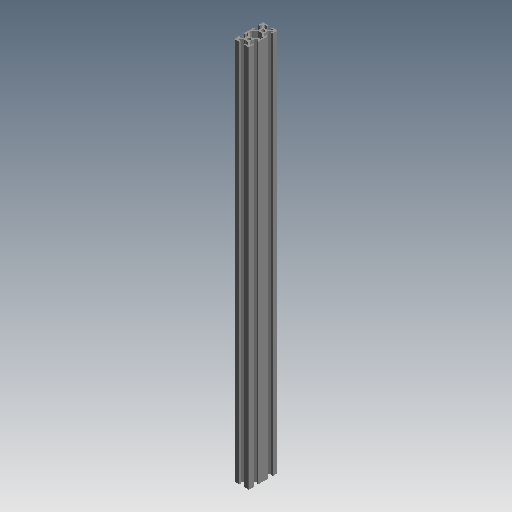
# Autodesk Inventor part: HFS5-2040-530
Saved by Autodesk Inventor 2020 (Build 240168000, 168)
## iProperties
Part Number: HFS5-2040-530
Material: Generic
Catalog Web Link: www.cadenas.de
Description: NFS5-2040, NFSB5-2040, HFS5-2040, HFSB5-2040, CAF5-2040, NFSF5-2040, HFSF5-2040-HFS5 Series Aluminum Extrusions 20,40 Square -2 Slots-
Vendor: MISUMI
Document SubType Name: Modeling
Designer: partserver
Manufacturer: MISUMI
Mass: 171.584 g
Surface Area: 1671.65 cm^2
Volume: 171.584 cm^3
Density: 1 g/cm^3
Appearance: PSOLRGB-175-175-175
Category: PARTsolutions
Company: MISUMI
Title: HFS5-2040-530
Author: Cadenas PARTsolutions
Comments: HFS5 Series Aluminum Extrusions 20,40 Square -2 Slots-
Autodesk Inventor part; units mm, degrees
sketch "Sketch_1" plane through (0, 0, 0) normal (0, 0, 1) x (1, 0, 0)
  line L0 (-10, -7) -> (-8, -7)
  line L1 (-8, -7) -> (-8, -4)
  line L2 (-8, -4) -> (-7.0607, -4)
  line L3 (-7.0607, -4) -> (-4, -7.0607)
  line L4 (-4, -7.0607) -> (-4, -9.4804)
  line L5 (-4, -9.4804) -> (-3.7, -10)
  line L6 (-3.7, -10) -> (-4, -10.5196)
  line L7 (-4, -10.5196) -> (-4, -12.9393)
  line L8 (-4, -12.9393) -> (-7.0607, -16)
  line L9 (-7.0607, -16) -> (-8, -16)
  line L10 (-8, -16) -> (-8, -13)
  line L11 (-8, -13) -> (-10, -13)
  line L12 (-10, -13) -> (-10, -19)
  arc A0 (-10, -19) -> (-9, -20) centre (-9, -19) ccw
  line L13 (-9, -20) -> (-3, -20)
  line L14 (-3, -20) -> (-3, -18)
  line L15 (-3, -18) -> (-6, -18)
  line L16 (-6, -18) -> (-6, -17.0607)
  line L17 (-6, -17.0607) -> (-2.9393, -14)
  line L18 (-2.9393, -14) -> (-0.5196, -14)
  line L19 (-0.5196, -14) -> (0, -13.7)
  line L20 (0, -13.7) -> (0.5196, -14)
  line L21 (0.5196, -14) -> (2.9393, -14)
  line L22 (2.9393, -14) -> (6, -17.0607)
  line L23 (6, -17.0607) -> (6, -18)
  line L24 (6, -18) -> (3, -18)
  line L25 (3, -18) -> (3, -20)
  line L26 (3, -20) -> (9, -20)
  arc A1 (9, -20) -> (10, -19) centre (9, -19) ccw
  line L27 (10, -19) -> (10, -13)
  line L28 (10, -13) -> (8, -13)
  line L29 (8, -13) -> (8, -16)
  line L30 (8, -16) -> (7.0607, -16)
  line L31 (7.0607, -16) -> (4, -12.9393)
  line L32 (4, -12.9393) -> (4, -10.5196)
  line L33 (4, -10.5196) -> (3.7, -10)
  line L34 (3.7, -10) -> (4, -9.4804)
  line L35 (4, -9.4804) -> (4, -7.0607)
  line L36 (4, -7.0607) -> (7.0607, -4)
  line L37 (7.0607, -4) -> (8, -4)
  line L38 (8, -4) -> (8, -7)
  line L39 (8, -7) -> (10, -7)
  line L40 (10, -7) -> (10, 7)
  line L41 (10, 7) -> (8, 7)
  line L42 (8, 7) -> (8, 4)
  line L43 (8, 4) -> (7.0607, 4)
  line L44 (7.0607, 4) -> (4, 7.0607)
  line L45 (4, 7.0607) -> (4, 9.4804)
  line L46 (4, 9.4804) -> (3.7, 10)
  line L47 (3.7, 10) -> (4, 10.5196)
  line L48 (4, 10.5196) -> (4, 12.9393)
  line L49 (4, 12.9393) -> (7.0607, 16)
  line L50 (7.0607, 16) -> (8, 16)
  line L51 (8, 16) -> (8, 13)
  line L52 (8, 13) -> (10, 13)
  line L53 (10, 13) -> (10, 19)
  arc A2 (10, 19) -> (9, 20) centre (9, 19) ccw
  line L54 (9, 20) -> (3, 20)
  line L55 (3, 20) -> (3, 18)
  line L56 (3, 18) -> (6, 18)
  line L57 (6, 18) -> (6, 17.0607)
  line L58 (6, 17.0607) -> (2.9393, 14)
  line L59 (2.9393, 14) -> (0.5196, 14)
  line L60 (0.5196, 14) -> (0, 13.7)
  line L61 (0, 13.7) -> (-0.5196, 14)
  line L62 (-0.5196, 14) -> (-2.9393, 14)
  line L63 (-2.9393, 14) -> (-6, 17.0607)
  line L64 (-6, 17.0607) -> (-6, 18)
  line L65 (-6, 18) -> (-3, 18)
  line L66 (-3, 18) -> (-3, 20)
  line L67 (-3, 20) -> (-9, 20)
  arc A3 (-9, 20) -> (-10, 19) centre (-9, 19) ccw
  line L68 (-10, 19) -> (-10, 13)
  line L69 (-10, 13) -> (-8, 13)
  line L70 (-8, 13) -> (-8, 16)
  line L71 (-8, 16) -> (-7.0607, 16)
  line L72 (-7.0607, 16) -> (-4, 12.9393)
  line L73 (-4, 12.9393) -> (-4, 10.5196)
  line L74 (-4, 10.5196) -> (-3.7, 10)
  line L75 (-3.7, 10) -> (-4, 9.4804)
  line L76 (-4, 9.4804) -> (-4, 7.0607)
  line L77 (-4, 7.0607) -> (-7.0607, 4)
  line L78 (-7.0607, 4) -> (-8, 4)
  line L79 (-8, 4) -> (-8, 7)
  line L80 (-8, 7) -> (-10, 7)
  line L81 (-10, 7) -> (-10, -7)
  line L82 (-8, 1.7) -> (-8, -1.7)
  arc A4 (-8, -1.7) -> (-7.7, -2) centre (-7.7, -1.7) ccw
  line L83 (-7.7, -2) -> (-7.0636, -2)
  arc A5 (-6.8515, -2.0879) -> (-7.0636, -2) centre (-7.0636, -2.3) ccw
  line L84 (-6.8515, -2.0879) -> (-2.9393, -6)
  line L85 (-2.9393, -6) -> (2.9393, -6)
  line L86 (2.9393, -6) -> (6.8515, -2.0879)
  arc A6 (7.0636, -2) -> (6.8515, -2.0879) centre (7.0636, -2.3) ccw
  line L87 (7.0636, -2) -> (7.7, -2)
  arc A7 (7.7, -2) -> (8, -1.7) centre (7.7, -1.7) ccw
  line L88 (8, -1.7) -> (8, 1.7)
  arc A8 (8, 1.7) -> (7.7, 2) centre (7.7, 1.7) ccw
  line L89 (7.7, 2) -> (7.0636, 2)
  arc A9 (6.8515, 2.0879) -> (7.0636, 2) centre (7.0636, 2.3) ccw
  line L90 (6.8515, 2.0879) -> (2.9393, 6)
  line L91 (2.9393, 6) -> (-2.9393, 6)
  line L92 (-2.9393, 6) -> (-6.8515, 2.0879)
  arc A10 (-7.0636, 2) -> (-6.8515, 2.0879) centre (-7.0636, 2.3) ccw
  line L93 (-7.0636, 2) -> (-7.7, 2)
  arc A11 (-7.7, 2) -> (-8, 1.7) centre (-7.7, 1.7) ccw
  constraints: 188 end point, 24 point on circle, 12 centre point
extrude "Extrusion1" add sketch "Sketch_1" against normal blind 530
sketch "Sketch2" plane through (0, 0, -530) normal (0, 0, -1) x (-1, 0, 0)
  point P0 (0, 10)
hole "Hole1" at (0, 10, -530) direction (0, 0, 1) diameter 4.2 depth 530
pattern_linear "Rectangular Pattern1" count 2 spacing 20 along (0, -1, 0) of "Hole1"
ref_plane "C1_XY" through (0, 0, 0) normal (0, 0, 1) x (1, 0, 0)
ref_plane "C1_YZ" through (0, 0, 0) normal (1, 0, 0) x (0, 1, 0)
ref_plane "C1_ZX" through (0, 0, 0) normal (0, 1, 0) x (0, 0, 1)
body "Solid1"
